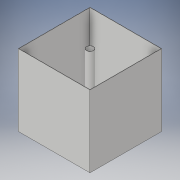
# Autodesk Inventor part: sebis-1
Saved by Autodesk Inventor 2019.1 (Build 231200000, 200)
## iProperties
Created: 2018-12-18
Part Number: sebis-1
Material: 一般
Document SubType Name: Modeling
Designer: Masaya
Density: 1 g/cm^3
Appearance: 既定
Author: Masaya
Autodesk Inventor part; units mm, degrees
ref_plane "YZ Plane" through (0, 0, 0) normal (1, 0, 0) x (0, 1, 0)
ref_plane "XZ Plane" through (0, 0, 0) normal (0, 1, 0) x (-1, 0, 0)
ref_plane "XY Plane" through (0, 0, 0) normal (0, 0, 1) x (1, 0, 0)
sketch "スケッチ1" plane through (0, 0, 0) normal (0, 1, 0) x (-1, 0, 0)
  line L0 (0, 0) -> (1010, 0)
  line L1 (1010, 0) -> (1010, 1010)
  line L2 (1010, 1010) -> (0, 1010)
  line L3 (0, 1010) -> (0, 0)
  dimension "d0" = 1010
  dimension "d1" = 1010
  constraints: 8 end point, 2 parallel, 1 horizontal, 1 perpendicular
  measures "d0" distance of L1.end L2.end
  measures "d1" distance of L0.end L1.end
extrude "押し出し1" add sketch "スケッチ1" along normal blind 10
sketch "スケッチ2" plane through (0, 10, 0) normal (0, 1, 0) x (1, 0, 0)
  line L0 (-1005, -1005) -> (-5, -1005)
  line L1 (-5, -1005) -> (-5, -5)
  line L2 (-5, -5) -> (-1005, -5)
  line L3 (-1005, -5) -> (-1005, -1005)
  line L4 (-1010, 0) -> (-1010, -1010) projected
  line L5 (-1010, -1010) -> (0, -1010) projected
  line L6 (0, 0) -> (-1010, 0) projected
  line L7 (-1010, 0) -> (-1010, -1010) projected
  line L8 (-1010, -1010) -> (0, -1010) projected
  line L9 (0, -1010) -> (0, 0) projected
  dimension "d4" = 1000
  dimension "d5" = 1000
  dimension "d6" = 5
  dimension "d7" = 5
  constraints: 8 end point, 2 parallel, 1 horizontal, 1 perpendicular
  measures "d4" distance of L2.end L1.end
  measures "d5" distance of L1.end L0.end
  measures "d6" distance between parallel lines of L3 L4
  measures "d7" distance between parallel lines of L0 L5
extrude "押し出し2" add sketch "スケッチ2" along normal blind 1000
sketch "スケッチ3" plane through (0, 10, 0) normal (0, 1, 0) x (1, 0, 0)
  circle A0 centre (-505, -505) radius 50
  line L0 (-1005, -1005) -> (-1005, -5) projected
  line L1 (-5, -1005) -> (-1005, -1005) projected
  circle A1 centre (-505, -505) radius 47.5
  point P0 (0, 0)
  dimension "d10" = 100
  dimension "d11" = 500
  dimension "d12" = 500
  dimension "d13" = 95
  constraints: 2 centre point, 1 coincident
  measures "d10" diameter of A0
  measures "d11" distance from line of L0 A0.centre
  measures "d12" distance from line of L1 A0.centre
  measures "d13" diameter of A1
extrude "押し出し3" add sketch "スケッチ3" along normal blind 1000
